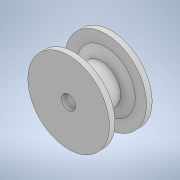
# Autodesk Inventor part: updated_wheel
Saved by Autodesk Inventor 2022 (Build 260153000, 153)
## iProperties
Created: 2023-03-03
Part Number: updated_wheel
Material: Generic
Document SubType Name: Modeling
Designer: matia
Density: 1 g/cm^3
Appearance: Default
Author: matia
Autodesk Inventor part; units mm, degrees
ref_plane "YZ Plane" through (0, 0, 0) normal (1, 0, 0) x (0, 1, 0)
ref_plane "XZ Plane" through (0, 0, 0) normal (0, 1, 0) x (-1, 0, 0)
ref_plane "XY Plane" through (0, 0, 0) normal (0, 0, 1) x (1, 0, 0)
sketch "Sketch1" plane through (0, 0, 0) normal (0, 1, 0) x (-1, 0, 0)
  line L0 (0, 0) -> (0, -4.826)
  line L1 (0, -4.826) -> (0, 0)
  line L2 (0, 0) -> (0, 4.826)
  line L3 (0, 4.826) -> (9.1948, 4.826)
  line L4 (9.1948, -4.826) -> (0, -4.826)
  line L5 (9.1948, 4.826) -> (9.1948, 3.556)
  line L6 (9.1948, 3.556) -> (6.6548, 3.556)
  line L7 (9.1948, -4.826) -> (9.1948, -3.556)
  line L8 (9.1948, -3.556) -> (6.6548, -3.556)
  line L9 (9.1948, 4.826) -> (9.1948, 3.556)
  line L10 (9.1948, -3.556) -> (9.1948, -4.826)
  line L11 (9.1948, 0) -> (6.0198, 0)
  line L12 (5.6388, 0) -> (4.3688, 0)
  line L13 (4.3688, 0) -> (4.3688, -2.54)
  line L14 (4.3688, -2.54) -> (4.3688, 0)
  line L15 (4.3688, 0) -> (4.3688, 2.54)
  line L16 (4.3688, 2.54) -> (6.6548, 3.556)
  line L17 (4.3688, -2.54) -> (6.6548, -3.556)
  dimension "d0" = 4.826
  dimension "d1" = 4.826
  dimension "d2" = 9.1948
  dimension "d3" = 1.27
  dimension "d4" = 2.54
  dimension "d5" = 1.27
  dimension "d6" = 2.54
  dimension "d7" = 3.175
  dimension "d9" = 1.27
  dimension "d10" = 2.54
  dimension "d11" = 2.54
  dimension "d12" = 2.54
  constraints: 36 end point, 8 perpendicular, 2 collinear, 2 horizontal, 2 point on line, 1 vertical
  measures "d0" distance of L0.start L0.end
  measures "d1" distance of L0.start L2.end
  measures "d2" distance of L2.end L3.end
  measures "d3" distance of L3.end L5.end
  measures "d4" distance of L5.end L6.end
  measures "d5" distance of L7.end L4.start
  measures "d6" distance of L7.end L8.end
  measures "d7" distance of L11.start L11.end
  measures "d9" distance of L12.start L12.end
  measures "d10" distance of L12.end L13.end
  measures "d11" distance of L13.end L12.end
  measures "d12" distance of L12.end L15.end
revolve "Revolution1" add sketch "Sketch1" angle 360 about axis through (0, 0, 0) along (0, 0, -1)
sketch "Sketch2" plane through (0, 0, -4.826) normal (0, 0, -1) x (-1, 0, 0)
  circle A0 centre (0, 0) radius 1.5875
  dimension "d14" = 3.175
  constraints: 1 centre point, 1 coincident
  measures "d14" diameter of A0
extrude "Extrusion1" cut sketch "Sketch2" against normal through all
body "Solid1"
